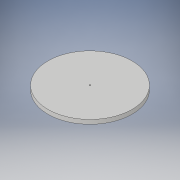
# Autodesk Inventor part: Rueda Superior
Saved by Autodesk Inventor 2017 (Build 210142000, 142)
## iProperties
Created: 2017-01-19
Part Number: Rueda Superior
Material: Generic
Document SubType Name: Modeling
Designer: A. Matías Quezada
Density: 1 g/cm^3
Appearance: Default
Author: A. Matías Quezada
Autodesk Inventor part; units mm, degrees
ref_plane "YZ Plane" through (0, 0, 0) normal (1, 0, 0) x (0, 1, 0)
ref_plane "XZ Plane" through (0, 0, 0) normal (0, 1, 0) x (-1, 0, 0)
ref_plane "XY Plane" through (0, 0, 0) normal (0, 0, 1) x (1, 0, 0)
sketch "Sketch1" plane through (0, 0, 0) normal (0, 0, 1) x (1, 0, 0)
  circle A0 centre (0, 0) radius 30
  dimension "d0" = 60
  constraints: 1 centre point, 1 coincident
  measures "d0" diameter of A0
extrude "Extrusion1" add sketch "Sketch1" along normal blind 3
sketch "Sketch2" plane through (0, 0, 0) normal (0, 0, -1) x (-1, 0, 0)
  arc A0 (0, 12) -> (0, -18) centre (0, -3) ccw
  arc A1 (0, -12) -> (0, 18) centre (0, 3) ccw
  circle A2 centre (0, 0) radius 30 projected
  line L0 (0, -18) -> (0, -12)
  line L1 (0, 12) -> (0, 18)
  dimension "d3" = 15
  dimension "d5" = 3
  dimension "d6" = 3
  constraints: 4 end point, 4 point on circle, 2 centre point, 2 collinear, 1 equal radius, 1 vertical
  measures "d3" radius of A0
  measures "d5" distance of A0.centre point (0, 0)
  measures "d6" distance of A1.centre point (0, 0)
extrude "Extrusion2" add sketch "Sketch2" along normal blind 3 contours L1 A1 L0 A0
sketch "Sketch3" plane through (0, 0, 3) normal (0, 0, 1) x (1, 0, 0)
  point P0 (0, 0)
  point P1 (0, 0)
  constraints: 1 coincident
hole "Hole1" at (0, 0, 3) direction (0, 0, -1) diameter 1 end through all
equation "\"d0\" = rs_diametro"
equation "\"d1\" = rs_grosor"
equation "\"d3\" = 0.5 * rs_gancho_diametro"
equation "\"d5\" = rs_gancho_diente"
equation "\"d6\" = rs_gancho_diente"
equation "\"d7\" = rs_gancho_grosor"
equation "\"d9\" = ri_ancla_diametro"
equation "\"rs_diametro\" = 60"
equation "\"rs_grosor\" = 3"
equation "\"rs_gancho_diametro\" = 30"
equation "\"rs_gancho_grosor\" = 3"
equation "\"ri_ancla_diametro\" = 1"
equation "\"rs_gancho_diente\" = 3"
body "Solid1"
